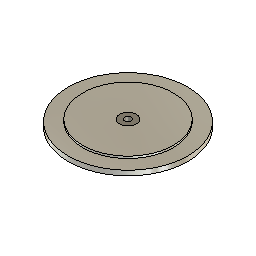
Top Rotary Disk v14 (Autodesk Fusion 360 design; units mm, degrees)
Autodesk Fusion 360 part; units mm, degrees
sketch "Sketch1" plane through (0, 0, 0) normal (0, 0, 1) x (1, 0, 0)
  circle A0 centre (0, 0) radius 89
  circle A1 centre (0, 0) radius 67.55
  dimension "d1" = 178
  dimension "d2" = 135.1
  constraint coincident A0.centre A1.centre
  measures "d1" diameter of A0
  measures "d2" diameter of A1
extrude "Extrude1" add sketch "Sketch1" along normal blind 8 contours A1 makes body 1
extrude "Extrude2" add sketch "Sketch1" along normal blind 5 bodies 1
sketch "Sketch2" plane through (0, 0, 8) normal (0, 0, 1) x (-1, 0, 0)
  circle A0 centre (0, 0) radius 67.55
  circle A1 centre (0, 0) radius 12.5
  circle A2 centre (0, 0) radius 4.9
  dimension "d7" = 25
  dimension "d19" = 9.8
  constraint coincident A0.centre A1.centre
  measures "d7" diameter of A1
  measures "d19" diameter of A2
extrude "Extrude3" cut sketch "Sketch2" against normal blind 10 contours A1 | A2 bodies 1
sketch "Sketch3" plane through (0, 0, 0) normal (0, 0, 1) x (1, 0, 0)
  circle A0 centre (0, 0) radius 4.9
  circle A1 centre (0, 0) radius 12.5
  dimension "d10" = 9.8
  constraint coincident A0.centre A1.centre
  measures "d10" diameter of A0
extrude "Extrude5" add sketch "Sketch1" against normal blind 2.1882 contours A0 | A1 bodies 1
sketch "Sketch4" plane through (0, 0, -2.1882) normal (0, 0, -1) x (1, 0, 0)
  circle A0 centre (0, 0) radius 89
  circle A1 centre (0, 0) radius 19.05
  circle A2 centre (0, 0) radius 5.08
  dimension "d15" = 38.1
  dimension "d16" = 10.16
  constraint coincident A0.centre A1.centre
  measures "d15" diameter of A1
  measures "d16" diameter of A2
extrude "Extrude6" add sketch "Sketch4" along normal blind 12.7 contours A1 bodies 1
sketch "Sketch5" plane through (0, 0, 8) normal (0, 0, 1) x (-1, 0, 0)
  circle A0 centre (0, 0) radius 12.5
  circle A1 centre (0, 0) radius 4.9
extrude "Extrude7" add sketch "Sketch5" against normal up to surface (8 mm away) separate body makes body 2
equation "d13 = -( 0.283 in - 5 mm )"
named bodies: "Bearing"
